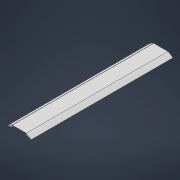
# Autodesk Inventor part: CeilingPanel
Saved by Autodesk Inventor 2021 (Build 250183000, 183)
## iProperties
Created: 2021-01-31
Part Number: CeilingPanel
Material: Generic
Document SubType Name: Modeling
Designer: argon
Density: 1 g/cm^3
Appearance: Default
Author: argon
Autodesk Inventor part; units mm, degrees
ref_plane "YZ Plane" through (0, 0, 0) normal (1, 0, 0) x (0, 1, 0)
ref_plane "XZ Plane" through (0, 0, 0) normal (0, 1, 0) x (-1, 0, 0)
ref_plane "XY Plane" through (0, 0, 0) normal (0, 0, 1) x (1, 0, 0)
sketch "Sketch1" plane through (0, 0, 0) normal (0, 0, 1) x (1, 0, 0)
  circle A0 centre (0, 0) radius 1750
  line L0 (-708.8723, 1600) -> (708.8723, 1600)
  line L1 (-695.1731, 1575) -> (695.1731, 1575)
  circle A1 centre (-745.4026, 1500) radius 75
  circle A2 centre (745.4026, 1500) radius 75
  line L2 (-723.4312, 1428.2905) -> (-1186.4179, 1286.4341)
  line L3 (723.4312, 1428.2905) -> (1186.4179, 1286.4341)
  line L4 (680.4507, 1537.5) -> (698.6372, 1569)
  line L5 (-680.4507, 1537.5) -> (-698.6372, 1569)
  arc A3 (-695.1731, 1575) -> (-698.6372, 1569) centre (-695.1731, 1571) ccw
  arc A4 (698.6372, 1569) -> (695.1731, 1575) centre (695.1731, 1571) ccw
  point P0 (-762.8073, 1575)
  point P1 (762.8073, 1575)
  dimension "d0" = 3500
  dimension "d1" = 1600
  dimension "d2" = 25
  dimension "d3" = 150
  dimension "d4" = 60
  dimension "d5" = 4
  constraints: 14 point on circle, 12 end point, 11 tangent, 5 centre point, 3 horizontal alignment, 2 equal radius, 2 horizontal, 2 point on line, 1 coincident
  measures "d0" diameter of A0
  measures "d1" distance from line of point (0, 0) L0
  measures "d2" distance between parallel lines of L1 L0
  measures "d3" diameter of A1
  measures "d4" angle of L5 L1
  measures "d5" radius of A3
extrude "Extrusion1" add sketch "Sketch1" along normal blind 14000 contours L3 A2 A0 | A0 A1 L2 | A2 L4 A4 L1 A3 L5 A1 A0 L0 | A2 | A1
sketch "Sketch2" plane through (0, 0, 14000) normal (0, 0, 1) x (1, 0, 0)
  line L0 (695.1731, 1575) -> (-695.1731, 1575)
  line L1 (-695.1731, 1575) -> (-695.1731, 1585)
  line L2 (-695.1731, 1585) -> (695.1731, 1585)
  line L3 (695.1731, 1585) -> (695.1731, 1575)
  point P0 (0, 0)
  dimension "d8" = 10
  constraints: 8 end point, 2 parallel, 1 coincident, 1 horizontal, 1 perpendicular
  measures "d8" distance of L0.end L1.end
extrude "Extrusion2" cut sketch "Sketch2" against normal through all
body "Solid1"
